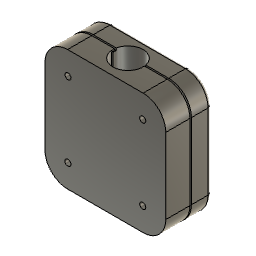
U6-LR pylväskiinnike v7 (Autodesk Fusion 360 design; units mm, degrees)
Autodesk Fusion 360 part; units mm, degrees
note: some values were not read from the file. Set by a fixed rule: which face or edge a step refers to.
sketch "Sketch1" plane through (0, 0, 0) normal (0, 1, 0) x (1, 0, 0)
  line L0 (15, 0) -> (65, 0)
  line L1 (80, -15) -> (80, -65)
  line L2 (65, -80) -> (15, -80)
  line L3 (0, -65) -> (0, -15)
  line L4 (40, -80) -> (40, 0)
  line L5 (0, -40) -> (80, -40)
  circle A0 centre (40, -40) radius 35 construction
  line L6 (80, -80) -> (0, 0) construction
  line L7 (0, -80) -> (80, 0) construction
  circle A1 centre (64.7487, -64.7487) radius 2
  circle A2 centre (64.7487, -15.2513) radius 2
  circle A3 centre (15.2513, -15.2513) radius 2
  circle A4 centre (15.2513, -64.7487) radius 2
  arc A5 (0, -65) -> (15, -80) centre (15, -65) ccw
  arc A6 (65, -80) -> (80, -65) centre (65, -65) ccw
  arc A7 (15, 0) -> (0, -15) centre (15, -15) ccw
  arc A8 (80, -15) -> (65, 0) centre (65, -15) ccw
  arc A9 (1, -65) -> (15, -79) centre (15, -65) ccw
  line L8 (65, -79) -> (15, -79)
  arc A10 (65, -79) -> (79, -65) centre (65, -65) ccw
  line L9 (79, -15) -> (79, -65)
  arc A11 (79, -15) -> (65, -1) centre (65, -15) ccw
  line L10 (15, -1) -> (65, -1)
  arc A12 (15, -1) -> (1, -15) centre (15, -15) ccw
  line L11 (1, -65) -> (1, -15)
  line L12 (65, -78.5) -> (15, -78.5)
  arc A13 (1.5, -65) -> (15, -78.5) centre (15, -65) ccw
  line L13 (1.5, -65) -> (1.5, -15)
  arc A14 (15, -1.5) -> (1.5, -15) centre (15, -15) ccw
  line L14 (15, -1.5) -> (65, -1.5)
  arc A15 (78.5, -15) -> (65, -1.5) centre (65, -15) ccw
  line L15 (78.5, -15) -> (78.5, -65)
  arc A16 (65, -78.5) -> (78.5, -65) centre (65, -65) ccw
  circle A17 centre (64.7487, -64.7487) radius 2.75
  circle A18 centre (64.7487, -15.2513) radius 2.75
  circle A19 centre (15.2513, -15.2513) radius 2.75
  circle A20 centre (15.2513, -64.7487) radius 2.75
  dimension "d5" = 80
  dimension "d6" = 80
  dimension "d13" = 70
  dimension "d14" = 4
  dimension "d16" = 360
  dimension "d22" = 15
  dimension "d23" = 15
  dimension "d24" = 15
  dimension "d25" = 15
  dimension "d28" = 1
  dimension "d42" = -1.5
  dimension "d48" = 5.5
  dimension "d50" = 360
  constraint horizontal L0
  constraint vertical L1
  constraint horizontal L2
  constraint vertical L3
  constraint coincident L6.end origin
  constraint midpoint L4 A0.centre
  constraint coincident A0 A1.centre
  constraint coincident L6 A1.centre
  constraint coincident L2 L4.start
  constraint coincident L3 L5.start
  constraint coincident L7.start L2
  constraint coincident L7.start L3
  constraint tangent L2 A5
  constraint tangent L3 A5
  constraint coincident L1 L5.end
  constraint coincident L6.start L2
  constraint coincident L6.start L1
  constraint tangent L2 A6
  constraint tangent L1 A6
  constraint coincident L0 L4.end
  constraint coincident L6.end L3
  constraint coincident L6.end L0
  constraint tangent L3 A7
  constraint tangent L0 A7
  constraint coincident L7.end L0
  constraint coincident L7.end L1
  constraint tangent L0 A8
  constraint tangent L1 A8
  constraint concentric A1 A17
  measures "d5" distance of L6.end L7.end
  measures "d6" distance of L6.end L7.start
  measures "d13" diameter of A0
  measures "d14" diameter of A1
  measures "d22" radius of A5
  measures "d23" radius of A6
  measures "d24" radius of A7
  measures "d25" radius of A8
  measures "d48" diameter of A17
extrude "Extrude1" add sketch "Sketch1" along normal blind 30 contours L0 L3 L4 L5 A7 L10 A12 L11 | L0 L1 L4 L5 A8 L9 A11 L10 | L4 L5 L9 A11 L10 L14 A15 L15 | L4 L5 L10 A12 L11 L13 A14 L14 | L2 L3 L4 L5 A5 A9 L8 L11 | L4 L5 L14 A15 L15 | L4 L5 L13 A14 L14 | L4 L5 A9 L8 L11 L12 A13 L13 | L1 L2 L4 L5 A6 L8 A10 L9 | L4 L5 L12 L15 A16 | L4 L5 L12 A13 L13 | L4 L5 L8 A10 L9 L12 L15 A16 | A1 | A2 | A3 | A4 | A17 | A18 | A19 | A20 makes body 1
sketch "Sketch2" plane through (0, 0, 80) normal (0, 0, 1) x (-1, 0, 0)
  line L0 (-15, 0) -> (-65, 0)
  line L1 (-65, -30) -> (-15, -30)
  line L2 (0, -20) -> (-80, -20)
  line L3 (-40, -30) -> (-40, 0)
  circle A0 centre (-40, -15) radius 10
  line L4 (-65, 0) -> (-65, -30)
  line L5 (-15, -30) -> (-15, 0)
  dimension "d9" = 20
  constraint midpoint L1 L3.start
  constraint midpoint L0 L3.end
  constraint midpoint L3 A0.centre
  measures "d9" diameter of A0
extrude "Extrude2" cut sketch "Sketch2" against normal up to surface (80 mm away) contours L2 L3 A0 | L2 L3 A0 | L2 L3 A0 | L2 L3 A0 bodies 1
extrude "Extrude3" cut sketch "Sketch1" along normal up to surface (30 mm away) contours A1 | A2 | A3 | A4 bodies 1
ref_plane "WorkPlane1" through (40, 14.9928, 80) normal (0, -1, 0) x (1, 0, 0)
split "Split1" by plane through (40, 14.9928, 80) normal (0, -1, 0) bodies 1 makes body 2 at (32.2391, 0, 47.7961)
extrude "Extrude4" cut sketch "Sketch1" along normal blind 2 from surface at 14.9928 contours L0 L3 L4 L5 A7 L10 A12 L11 | L0 L1 L4 L5 A8 L9 A11 L10 | L2 L3 L4 L5 A5 A9 L8 L11 | L1 L2 L4 L5 A6 L8 A10 L9 bodies 1
extrude "Extrude5" add sketch "Sketch1" along normal blind 1 from surface at 14.9928 contours L0 L3 L4 L5 A7 L10 A12 L11 | L0 L1 L4 L5 A8 L9 A11 L10 | L2 L3 L4 L5 A5 A9 L8 L11 | L1 L2 L4 L5 A6 L8 A10 L9 bodies 2
extrude "Extrude6" cut sketch "Sketch1" against normal blind 1 from surface at 14.9928 contours L4 L5 L9 A11 L10 L14 A15 L15 | L4 L5 L10 A12 L11 L13 A14 L14 | L4 L5 L14 A15 L15 | L4 L5 L13 A14 L14 | L4 L5 A9 L8 L11 L12 A13 L13 | L4 L5 L12 L15 A16 | L4 L5 L12 A13 L13 | L4 L5 L8 A10 L9 L12 L15 A16 | A17 | A18 | A19 | A20 bodies 2
extrude "Extrude7" cut sketch "Sketch2" against normal up to surface (80 mm away) contours L2 L3 A0 | L2 L3 A0 | L2 L3 A0 | L2 L3 A0 bodies 2
extrude "Extrude8" cut sketch "Sketch1" along normal blind 2 from surface at 14.9928 contours L4 L5 L9 A11 L10 L14 A15 L15 | L4 L5 L10 A12 L11 L13 A14 L14 | L4 L5 A9 L8 L11 L12 A13 L13 | L4 L5 L8 A10 L9 L12 L15 A16 bodies 1
extrude "Extrude9" add sketch "Sketch1" along normal up to surface (15.0072 mm away) from surface at 14.9928 contours A1 | A2 | A3 | A4 bodies 1
extrude "Extrude10" cut sketch "Sketch1" along normal blind 8 from surface at 14.9928 contours A1 | A2 | A3 | A4 | A17 | A18 | A19 | A20 bodies 1
fillet "Fillet1" radius 2 8 edges at (80, 30, 40) (75.6066, 30, 4.3934) (40, 30, 0) (4.3934, 30, 4.3934) (0, 30, 40) (4.3934, 30, 75.6066) (40, 30, 80) (75.6066, 30, 75.6066) on bodies 1
equation "blockWidth = 80 mm"
equation "blockHeight = 80 mm"
equation "blockThickness = 30 mm"
equation "tubeDiameter = 20 mm"
equation "d5 = blockWidth"
equation "d6 = blockHeight"
equation "d7 = blockThickness"
equation "d9 = tubeDiameter"
equation "plateHoleDistance = 70 mm"
equation "plateHoleDiameter = 4 mm"
equation "d13 = plateHoleDistance"
equation "d14 = plateHoleDiameter"
equation "d22 = blockFillet"
equation "d23 = blockFillet"
equation "d24 = blockFillet"
equation "d25 = blockFillet"
equation "blockFillet = 15 mm"
equation "blockLipWidth = 1 mm"
equation "d28 = blockLipWidth"
equation "blockLipDepth = 1 mm"
equation "d31 = 2 * blockLipDepth"
equation "d34 = blockLipDepth"
equation "d37 = -blockLipDepth"
equation "d42 = -1.5 * blockLipWidth"
equation "d44 = 2 * blockLipDepth"
equation "heatInsertDiameter = 5.5 mm" comment "M4 brass heat insert"
equation "heatInsertLength = 8 mm" comment "M4 brass heat insert"
equation "d48 = heatInsertDiameter"
equation "d55 = heatInsertLength"
named bodies: "Takapuolisko", "Etupuolisko"
